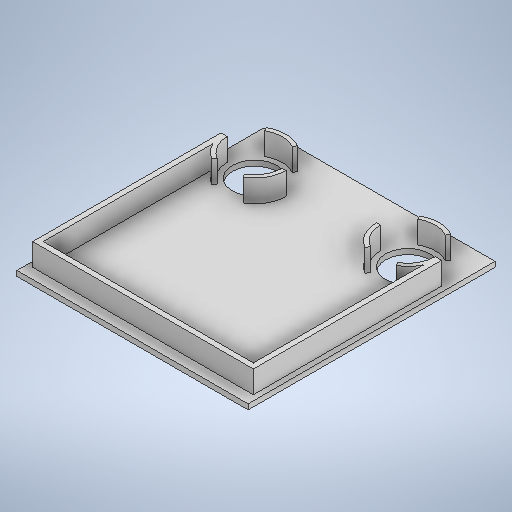
# Autodesk Inventor part: case_v1.1
Saved by Autodesk Inventor 2025 (Build 290162000, 162)
## iProperties
Created: 2025-03-20
Part Number: case_v1.1
Material: Generic
Document SubType Name: Modeling
Designer: ethan
Density: 1 g/cm^3
Appearance: Default
Author: ethan
Autodesk Inventor part; units mm, degrees
ref_plane "YZ Plane" through (0, 0, 0) normal (1, 0, 0) x (0, 1, 0)
ref_plane "XZ Plane" through (0, 0, 0) normal (0, 1, 0) x (-1, 0, 0)
ref_plane "XY Plane" through (0, 0, 0) normal (0, 0, 1) x (1, 0, 0)
sketch "Sketch1" plane through (0, 0, 0) normal (0, 1, 0) x (-1, 0, 0)
  line L0 (0, 0) -> (-88, 0)
  line L1 (-88, 0) -> (-88, -94)
  line L2 (-88, -94) -> (0, -94)
  line L3 (0, -94) -> (0, 0)
  line L4 (0, -94) -> (0, -75.65)
  line L5 (0, -94) -> (-14.85, -94)
  circle A0 centre (-14.85, -75.65) radius 8.45
  line L6 (-44, -88.9444) -> (-44, -54.2543) construction
  circle A1 centre (-73.15, -75.65) radius 8.45
  dimension "d0" = 88
  dimension "d1" = 94
  dimension "d2" = 18.35
  dimension "d3" = 14.85
  dimension "d4" = 16.9
  dimension "d48" = 16.9
  constraints: 14 end point, 2 centre point, 2 parallel, 2 point on line, 1 horizontal, 1 perpendicular, 1 symmetric about line, 1 vertical, 1 other
  measures "d0" distance of L2.end L1.end
  measures "d1" distance of L1.end L0.end
  measures "d2" distance of L2.end L4.end
  measures "d3" distance of L2.end L5.end
  measures "d4" diameter of A0
  measures "d48" diameter of A1
extrude "Extrusion1" add sketch "Sketch1" along normal blind 2
sketch "Sketch3" plane through (0, 2, 0) normal (0, 1, 0) x (1, 0, 0)
  circle A0 centre (73.15, 75.65) radius 8.45 construction
  circle A1 centre (14.85, 75.65) radius 8.45 construction
  line L0 (0, 0) -> (4, 0) construction
  line L1 (4, 0) -> (4, 6) construction
  line L2 (4, 6) -> (0, 6) construction
  line L3 (0, 6) -> (0, 0) construction
  line L4 (88, 0) -> (84, 0) construction
  line L5 (84, 0) -> (84, 6) construction
  line L6 (84, 6) -> (88, 6) construction
  line L7 (88, 6) -> (88, 0) construction
  line L8 (4, 6) -> (2, 6) construction
  line L9 (2, 6) -> (2, 4) construction
  line L10 (2, 4) -> (4, 4) construction
  line L11 (4, 4) -> (4, 6) construction
  line L12 (2, 4) -> (6, 4)
  line L13 (6, 4) -> (6, 6)
  line L14 (6, 6) -> (2, 6)
  line L15 (2, 6) -> (2, 4)
  line L16 (2, 4) -> (4, 4)
  line L17 (4, 4) -> (4, 8)
  line L18 (4, 8) -> (2, 8)
  line L19 (2, 8) -> (2, 4)
  line L20 (86, 4) -> (82, 4)
  line L21 (82, 4) -> (82, 4)
  line L22 (82, 4) -> (86, 4)
  line L23 (86, 4) -> (86, 4)
  line L24 (86, 4) -> (84, 4)
  line L25 (84, 4) -> (84, 8)
  line L26 (84, 8) -> (86, 8)
  line L27 (86, 8) -> (86, 4)
  line L28 (44, 4.3599) -> (37, 4.3599) construction
  line L29 (88, -1) -> (0, -1) construction
  line L30 (37, -1) -> (51, -1) construction
  line L31 (51, -1) -> (51, 0) construction
  line L32 (51, 0) -> (37, 0) construction
  line L33 (37, 0) -> (37, -1) construction
  line L34 (37, -1) -> (51, -1)
  line L35 (51, -1) -> (51, 0)
  line L36 (51, 0) -> (37, 0)
  line L37 (37, 0) -> (37, -1)
  line L38 (0, 95) -> (88, 95) projected
  line L39 (37, 95) -> (51, 95)
  line L40 (51, 95) -> (51, 94)
  line L41 (51, 94) -> (37, 94)
  line L42 (37, 94) -> (37, 95)
  circle A2 centre (14.85, 75.65) radius 10.45
  circle A3 centre (14.85, 75.65) radius 11.95
  line L43 (14.85, 75.65) -> (26.8, 75.65) construction
  line L44 (14.85, 75.65) -> (20.825, 85.999) construction
  line L45 (14.85, 75.65) -> (8.875, 85.999) construction
  line L46 (14.85, 75.65) -> (2.9, 75.65) construction
  line L47 (14.85, 75.65) -> (8.875, 65.301) construction
  line L48 (14.85, 75.65) -> (20.825, 65.301) construction
  line L49 (9.625, 84.7) -> (8.875, 85.999) construction
  line L50 (9.625, 84.7) -> (8.875, 85.999)
  line L51 (20.825, 85.999) -> (20.075, 84.7)
  line L52 (25.3, 75.65) -> (26.8, 75.65)
  line L53 (20.825, 65.301) -> (20.075, 66.6)
  line L54 (9.625, 66.6) -> (8.875, 65.301)
  line L55 (4.4, 75.65) -> (2.9, 75.65)
  line L56 (44, 84.7433) -> (44, 74.6259) construction
  circle A4 centre (73.15, 75.65) radius 8.45 construction
  circle A5 centre (73.15, 75.65) radius 10.45
  circle A6 centre (73.15, 75.65) radius 11.95
  line L57 (73.15, 75.65) -> (61.2, 75.65) construction
  line L58 (73.15, 75.65) -> (67.175, 85.999) construction
  line L59 (73.15, 75.65) -> (79.125, 85.999) construction
  line L60 (73.15, 75.65) -> (85.1, 75.65) construction
  line L61 (73.15, 75.65) -> (79.125, 65.301) construction
  line L62 (73.15, 75.65) -> (67.175, 65.301) construction
  line L63 (78.375, 84.7) -> (79.125, 85.999) construction
  line L64 (78.375, 84.7) -> (79.125, 85.999)
  line L65 (67.175, 85.999) -> (67.925, 84.7)
  line L66 (62.7, 75.65) -> (61.2, 75.65)
  line L67 (67.175, 65.301) -> (67.925, 66.6)
  line L68 (78.375, 66.6) -> (79.125, 65.301)
  line L69 (83.6, 75.65) -> (85.1, 75.65)
  line L70 (86, 4) -> (82, 4)
  line L71 (82, 4) -> (82, 6)
  line L72 (82, 6) -> (86, 6)
  line L73 (86, 6) -> (86, 4)
  point P0 (2, 4)
  point P1 (4, 6)
  point P2 (84, 4)
  point P3 (67.175, 65.301)
  point P4 (79.125, 65.301)
  point P5 (2.9, 75.65)
  point P6 (8.875, 65.301)
  point P7 (20.825, 65.301)
  point P8 (84, 6)
  dimension "d11" = 4
  dimension "d12" = 6
  dimension "d13" = 4
  dimension "d14" = 6
  dimension "d15" = 2
  dimension "d16" = 2
  dimension "d17" = 4
  dimension "d18" = 4
  dimension "d19" = 4
  dimension "d20" = 2
  dimension "d21" = 4
  dimension "d22" = 7
  dimension "d23" = 14
  dimension "d24" = 14
  dimension "d25" = 1
  dimension "d26" = 2
  dimension "d27" = 1.5
  dimension "d30" = 360
  constraints: 144 end point, 21 parallel, 19 symmetric about line, 17 point on line, 16 point on circle, 11 perpendicular, 10 horizontal, 7 collinear, 5 centre point, 2 coincident, 1 vertical, 20 other
  measures "d11" distance of L2.end L1.end
  measures "d12" distance of L1.end L0.end
  measures "d13" distance of L5.end L6.end
  measures "d14" distance of L4.end L5.end
  measures "d15" distance of L10.end L9.end
  measures "d16" distance of L9.end L8.end
  measures "d17" distance of L14.end L13.end
  measures "d18" distance of L17.end L16.end
  measures "d19" distance of L21.end L22.end
  measures "d20" distance of L25.end L26.end
  measures "d21" distance of L24.end L25.end
  measures "d22" distance of L28.start L28.end
  measures "d23" distance of L30.start L30.end
  measures "d24" distance of L39.start L39.end
  measures "d25" distance of L39.end L40.end
  measures "d26" radial gap between concentric circles of A1 A2
  measures "d27" radial gap between concentric circles of A2 A3
extrude "Extrusion3" add sketch "Sketch3" along normal blind 8.5 contours L15 L14 L17 L12 | L17 L14 L13 L12 | L19 L18 L17 L14 | L20 L25 L72 L27 | L20 L71 L72 L25 | L72 L25 L26 L27 | L52 A3 L53 A2 | A2 L50 A3 L51 | L54 A3 L55 A2 | L69 A6 L68 A5 | A5 L65 A6 L64 | L67 A6 L66 A5
sketch "Sketch6" plane through (0, 2, 0) normal (0, 1, 0) x (1, 0, 0)
  arc A0 (78.375, 84.7) -> (67.925, 84.7) centre (73.15, 75.65) ccw construction
  line L0 (67.925, 84.7) -> (67.175, 85.999) construction
  arc A1 (79.125, 85.999) -> (67.175, 85.999) centre (73.15, 75.65) ccw construction
  line L1 (79.125, 85.999) -> (78.375, 84.7) construction
  line L2 (2, 8) -> (4, 8) construction
  line L3 (4, 8) -> (4, 6) construction
  line L4 (4, 6) -> (6, 6) construction
  line L5 (6, 6) -> (6, 4) construction
  line L6 (6, 4) -> (2, 4) construction
  line L7 (2, 4) -> (2, 8) construction
  line L8 (83.6, 75.65) -> (85.1, 75.65) construction
  arc A2 (79.125, 65.301) -> (85.1, 75.65) centre (73.15, 75.65) ccw construction
  line L9 (79.125, 65.301) -> (78.375, 66.6) construction
  arc A3 (78.375, 66.6) -> (83.6, 75.65) centre (73.15, 75.65) ccw construction
  line L10 (20.825, 85.999) -> (20.075, 84.7) construction
  arc A4 (20.075, 84.7) -> (9.625, 84.7) centre (14.85, 75.65) ccw construction
  line L11 (9.625, 84.7) -> (8.875, 85.999) construction
  arc A5 (20.825, 85.999) -> (8.875, 85.999) centre (14.85, 75.65) ccw construction
  line L12 (2.9, 75.65) -> (4.4, 75.65) construction
  arc A6 (4.4, 75.65) -> (9.625, 66.6) centre (14.85, 75.65) ccw construction
  line L13 (9.625, 66.6) -> (8.875, 65.301) construction
  arc A7 (2.9, 75.65) -> (8.875, 65.301) centre (14.85, 75.65) ccw construction
  line L14 (86, 8) -> (86, 4) construction
  line L15 (86, 4) -> (82, 4) construction
  line L16 (82, 4) -> (82, 6) construction
  line L17 (82, 6) -> (84, 6) construction
  line L18 (84, 6) -> (84, 8) construction
  line L19 (84, 8) -> (86, 8) construction
  arc A8 (62.7, 75.65) -> (67.925, 66.6) centre (73.15, 75.65) ccw construction
  line L20 (67.925, 66.6) -> (67.175, 65.301) construction
  arc A9 (61.2, 75.65) -> (67.175, 65.301) centre (73.15, 75.65) ccw construction
  line L21 (61.2, 75.65) -> (62.7, 75.65) construction
  line L22 (25.3, 75.65) -> (26.8, 75.65) construction
  arc A10 (20.825, 65.301) -> (26.8, 75.65) centre (14.85, 75.65) ccw construction
  line L23 (20.825, 65.301) -> (20.075, 66.6) construction
  arc A11 (20.075, 66.6) -> (25.3, 75.65) centre (14.85, 75.65) ccw construction
  line L24 (88, 94) -> (0, 94) construction
  line L25 (0, 94) -> (0, 0) construction
  line L26 (0, 0) -> (88, 0) construction
  line L27 (88, 0) -> (88, 94) construction
  circle A12 centre (73.15, 75.65) radius 8.45 construction
  circle A13 centre (14.85, 75.65) radius 8.45 construction
  line L28 (6, 4) -> (82, 4) construction
  line L29 (82, 4) -> (82, 6) construction
  line L30 (82, 6) -> (6, 6) construction
  line L31 (6, 6) -> (6, 4) construction
  line L32 (86, 8) -> (84, 8) construction
  line L33 (84, 8) -> (84, 75.65) construction
  line L34 (84, 75.65) -> (86, 75.65) construction
  line L35 (86, 75.65) -> (86, 8) construction
  line L36 (2, 8) -> (4, 8) construction
  line L37 (4, 8) -> (4, 75.65) construction
  line L38 (4, 75.65) -> (2, 75.65) construction
  line L39 (2, 75.65) -> (2, 8) construction
  line L40 (2, 75.65) -> (4, 75.65)
  line L41 (4, 75.65) -> (4, 8)
  line L42 (4, 8) -> (2, 8)
  line L43 (2, 8) -> (2, 75.65)
  line L44 (6, 6) -> (82, 6)
  line L45 (82, 6) -> (82, 4)
  line L46 (82, 4) -> (6, 4)
  line L47 (6, 4) -> (6, 6)
  line L48 (84, 8) -> (86, 8)
  line L49 (86, 8) -> (86, 75.65)
  line L50 (86, 75.65) -> (84, 75.65)
  line L51 (84, 75.65) -> (84, 8)
  dimension "d44" = 2
  dimension "d45" = 2
  constraints: 48 end point, 12 parallel, 6 horizontal, 6 perpendicular, 2 point on line
  measures "d44" distance of L33.end L34.end
  measures "d45" distance of L38.end L37.end
extrude "Extrusion6" add sketch "Sketch6" along normal blind 8.5
body "Solid1"
